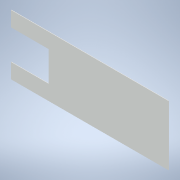
# Autodesk Inventor part: plexiglass2
Saved by Autodesk Inventor 2021 (Build 250183000, 183)
## iProperties
Created: 2021-03-23
Part Number: plexiglass2
Material: Generic
Document SubType Name: Modeling
Designer: con_c_000
Density: 1 g/cm^3
Appearance: Default
Author: con_c_000
Autodesk Inventor part; units mm, degrees
ref_plane "YZ Plane" through (0, 0, 0) normal (1, 0, 0) x (0, 1, 0)
ref_plane "XZ Plane" through (0, 0, 0) normal (0, 1, 0) x (-1, 0, 0)
ref_plane "XY Plane" through (0, 0, 0) normal (0, 0, 1) x (1, 0, 0)
sketch "Sketch1" plane through (0, 0, 0) normal (0, 0, 1) x (1, 0, 0)
  line L0 (-116.7504, -3.6908) -> (-895.8037, -3.6908)
  line L1 (-895.8037, -3.6908) -> (-895.8037, 301.1092)
  line L2 (-895.8037, 301.1092) -> (-116.7504, 301.1092)
  line L3 (-116.7504, 301.1092) -> (-116.7504, -3.6908)
  line L4 (-895.8037, -3.6908) -> (-944.7633, -3.6908)
  line L5 (-944.7633, -3.6908) -> (-944.7633, 72.5092)
  line L6 (-944.7633, 72.5092) -> (-895.8037, 72.5092)
  line L7 (-895.8037, 72.5092) -> (-895.8037, -3.6908)
  line L8 (-895.8037, 301.1092) -> (-944.7633, 301.1092)
  line L9 (-944.7633, 301.1092) -> (-944.7633, 224.9092)
  line L10 (-944.7633, 224.9092) -> (-895.8037, 224.9092)
  line L11 (-895.8037, 224.9092) -> (-895.8037, 301.1092)
  line L12 (-116.5344, 301.1092) -> (-116.5344, -3.6908) projected
  point P0 (0, 0)
  dimension "d1" = 304.8
  dimension "d4" = 76.2
  dimension "d5" = 76.2
  constraints: 24 end point, 6 parallel, 3 horizontal, 3 perpendicular, 1 point on line
  measures "d1" distance of L0.end L1.end
  measures "d4" distance of L4.end L5.end
  measures "d5" distance of L9.end L8.end
extrude "Extrusion1" add sketch "Sketch1" along normal blind 2.54
body "Solid1"
